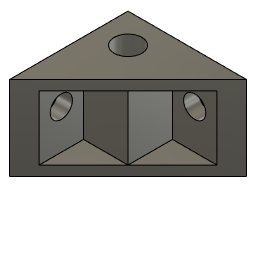
equerre v5 (Autodesk Fusion 360 design; units mm, degrees)
Autodesk Fusion 360 part; units mm, degrees
sketch "Sketch1" plane through (0, 0, 0) normal (0, 1, 0) x (1, 0, 0)
  line L0 (0, 0) -> (24, 0)
  line L1 (0, 0) -> (0, -24)
  circle A0 centre (6, -6) radius 2.8
  line L2 (0, -24) -> (24, 0)
  line L3 (0, 0) -> (12, 0)
  line L4 (12, 0) -> (12, -12)
  line L5 (12, -12) -> (0, -12)
  line L6 (0, -12) -> (0, 0)
  line L7 (3, 0) -> (3, -23)
  line L8 (3, -3) -> (21, -3)
  dimension "d3" = 5.6
  dimension "d4" = 6
  dimension "d5" = 6
  dimension "d6" = 12
  dimension "d7" = 12
  dimension "d14" = 3
  dimension "d15" = 3
  constraint coincident L0.start L1.start
  constraint horizontal L0
  constraint perpendicular L0 L1
  constraint horizontal L3
  constraint vertical L4
  constraint horizontal L5
  constraint vertical L6
  constraint coincident L2 L4.end
  constraint coincident L0 L7.start
  constraint perpendicular L0 L7
  constraint coincident L7 L8.start
  constraint coincident L2 L8.end
  constraint perpendicular L7 L8
  measures "d3" diameter of A0
  measures "d4" distance of L1 A0.centre
  measures "d5" distance of L0 A0.centre
  measures "d6" distance of L0.start L3.end
  measures "d7" distance of L0.start L5.end
  measures "d14" distance of L0 L8
  measures "d15" distance of L1 L7
extrude "Extrude1" add sketch "Sketch1" along normal blind 17 contours L0 L1 L3 L5 L6 L7 | L0 L3 L4 L7 L8 | L4 L5 L7 L8
extrude "Extrude2" add sketch "Sketch1" along normal blind 2 contours L1 L2 L5 L7 | L0 L2 L4 L8 | L2 L5 L7 | L2 L4 L8
extrude "Extrude3" add sketch "Sketch1" along normal blind 17 contours L1 L2 L5 L7 | L0 L2 L4 L8
extrude "Extrude4" add sketch "Sketch1" against normal blind 2 from surface at 17 contours L2 L5 L7 | L2 L4 L8
sketch "Sketch2" plane through (0, 0, 3) normal (0, 0, 1) x (1, 0, 0)
  line L0 (21, 15) -> (12, 15)
  line L1 (12, 15) -> (12, 2)
  line L2 (12, 2) -> (21, 2)
  line L3 (21, 2) -> (21, 15)
  line L4 (12, 10) -> (21, 10) construction
  circle A0 centre (16.5, 10) radius 2.25
  point P0 (12, 10)
  point P1 (12, 8.5)
  dimension "d21" = 1.5
  dimension "d22" = 4.5
  constraint coincident L1 P0
  constraint midpoint L1 P1
  constraint coincident P0 L4.start
  constraint coincident L3 L4.end
  constraint perpendicular L3 L4
  constraint midpoint L4 A0.centre
  measures "d21" distance of P0 P1
  measures "d22" diameter of A0
extrude "Extrude5" cut sketch "Sketch2" against normal through all contours A0
sketch "Sketch3" plane through (3, 0, 0) normal (1, 0, 0) x (0, 0, -1)
  line L0 (-12, 15) -> (-21, 15)
  line L1 (-21, 15) -> (-21, 2)
  line L2 (-21, 2) -> (-12, 2)
  line L3 (-12, 2) -> (-12, 15)
  line L4 (-12, 10) -> (-21, 10) construction
  circle A0 centre (-16.5, 10) radius 2.25
  point P0 (-12, 8.5)
  point P1 (-12, 10)
  dimension "d25" = 1.5
  dimension "d26" = 4.5
  constraint midpoint L3 P0
  constraint coincident L3 P1
  constraint coincident P1 L4.start
  constraint coincident L1 L4.end
  constraint perpendicular L1 L4
  constraint midpoint L4 A0.centre
  measures "d25" distance of P0 P1
  measures "d26" diameter of A0
extrude "Extrude6" cut sketch "Sketch3" against normal through all contours A0
equation "d8 = 20 mm - 3 mm"
named bodies: "equerre"
